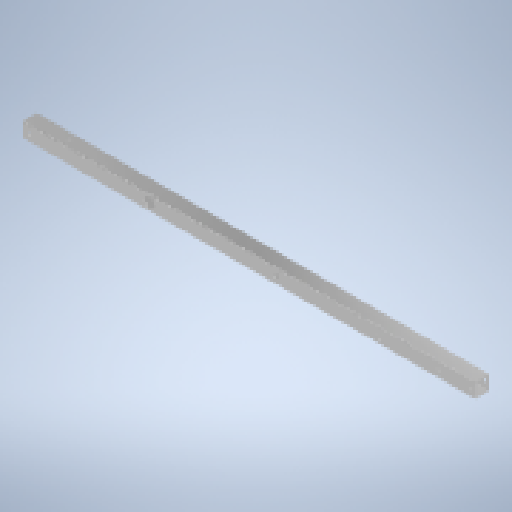
# Autodesk Inventor part: Längs_Traverse_vorne
Saved by Autodesk Inventor 2024.4 (Build 284460000, 460)
## iProperties
Created: 2026-01-10
Part Number: Längs_Traverse_vorne
Material: Aluminium 6061
Description: Längs_Traverse_vorne
Document SubType Name: Modeling
Designer: julia
Mass: 1006.1 g
Surface Area: 3721.63 cm^2
Volume: 372.629 cm^3
Density: 2.7 g/cm^3
Appearance: Aluminium - flach
DocNumber: Längs_Traverse_vorne.ipt
Folder: I60-Konstruktion\I60-Gruppe-7\Gestell\
VDS_Category: Konstruktion
Masse[kg]: 0,377 kg
Autodesk Inventor part; units mm, degrees
ref_plane "YZ Plane" through (0, 0, 0) normal (1, 0, 0) x (0, 1, 0)
ref_plane "XZ Plane" through (0, 0, 0) normal (0, 1, 0) x (-1, 0, 0)
ref_plane "XY Plane" through (0, 0, 0) normal (0, 0, 1) x (1, 0, 0)
sketch "Skizze1" plane through (0, 0, 0) normal (1, 0, 0) x (0, 1, 0)
  line L0 (-19, 20) -> (19, 20)
  line L1 (20, 19) -> (20, -19)
  line L2 (19, -20) -> (-19, -20)
  line L3 (-20, -19) -> (-20, 19)
  line L4 (-20, 20) -> (20, -20) construction
  line L5 (20, 20) -> (-20, -20) construction
  line L6 (-17.5, 18) -> (17.5, 18)
  line L7 (18, 17.5) -> (18, -17.5)
  line L8 (17.5, -18) -> (-17.5, -18)
  line L9 (-18, -17.5) -> (-18, 17.5)
  line L10 (-18, 18) -> (18, -18) construction
  line L11 (18, 18) -> (-18, -18) construction
  arc A0 (20, 19) -> (19, 20) centre (19, 19) ccw
  arc A1 (-19, 20) -> (-20, 19) centre (-19, 19) ccw
  arc A2 (-20, -19) -> (-19, -20) centre (-19, -19) ccw
  arc A3 (19, -20) -> (20, -19) centre (19, -19) ccw
  arc A4 (18, 17.5) -> (17.5, 18) centre (17.5, 17.5) ccw
  arc A5 (-17.5, 18) -> (-18, 17.5) centre (-17.5, 17.5) ccw
  arc A6 (17.5, -18) -> (18, -17.5) centre (17.5, -17.5) ccw
  arc A7 (-18, -17.5) -> (-17.5, -18) centre (-17.5, -17.5) ccw
  point P0 (0, 0)
  dimension "d0" = 40
  dimension "d1" = 40
  dimension "d2" = 36
  dimension "d3" = 36
  dimension "d4" = 1
  dimension "d5" = 0.5
  constraints: 24 end point, 16 point on circle, 16 point on line, 16 tangent, 8 centre point, 5 equal radius, 4 midpoint, 4 parallel, 2 horizontal, 2 perpendicular
  measures "d0" distance of L4.end L5.end
  measures "d1" distance of L5.start L4.end
  measures "d2" distance of L10.end L11.end
  measures "d3" distance of L11.start L10.end
  measures "d4" radius of A0
  measures "d5" radius of A4
extrude "Extrusion1" add sketch "Skizze1" along normal blind 1250
sketch "Skizze2" plane through (0, 20, 19) normal (0, 1, 0) x (1, 0, 0)
  line L0 (0, 19) -> (20, 19)
  line L1 (1250, 38) -> (1250, 0) projected
  line L2 (1250, 19) -> (1150, 19)
  circle A0 centre (1150, 19) radius 5.25
  circle A1 centre (20, 19) radius 5.25
  dimension "d9" = 20
  dimension "d10" = 100
  dimension "d11" = 10.5
  dimension "d12" = 10.5
  constraints: 4 end point, 2 centre point, 2 coincident, 2 horizontal, 1 midpoint
  measures "d9" distance of L0.start L0.end
  measures "d10" distance of L2.start L2.end
  measures "d11" diameter of A0
  measures "d12" diameter of A1
extrude "Extrusion2" cut sketch "Skizze2" against normal blind 1250
sketch "Skizze3" plane through (0, -19, 20) normal (0, 0, 1) x (1, 0, 0)
  line L0 (0, 19) -> (110, 19)
  line L1 (1250, 0) -> (1250, 38) projected
  line L2 (1250, 19) -> (1240, 19)
  circle A0 centre (110, 19) radius 3.2
  dimension "d15" = 110
  dimension "d18" = 6.4
  constraints: 4 end point, 2 horizontal, 1 centre point, 1 coincident, 1 midpoint
  measures "d15" distance of L0.start L0.end
  measures "d18" diameter of A0
extrude "Extrusion3" cut sketch "Skizze3" against normal blind 1250
sketch "Skizze4" plane through (0, -19, 20) normal (0, 0, 1) x (1, 0, 0)
  line L0 (0, 19) -> (110, 19)
  circle A0 centre (110, 19) radius 5.5
  dimension "d21" = 110
  dimension "d22" = 11
  constraints: 2 end point, 1 centre point, 1 coincident, 1 horizontal
  measures "d21" distance of L0.start L0.end
  measures "d22" diameter of A0
extrude "Extrusion4" cut sketch "Skizze4" against normal blind 2
sketch "Skizze6" plane through (0, -20, -19) normal (0, -1, 0) x (1, 0, 0)
  circle A0 centre (1150, 19) radius 5.25 projected
  line L0 (1150, 19) -> (350, 19)
  circle A1 centre (350, 19) radius 14
  point P0 (0, 19)
  dimension "d31" = 800
  dimension "d32" = 28
  constraints: 2 end point, 1 centre point, 1 coincident, 1 horizontal
  measures "d31" distance of L0.start L0.end
  measures "d32" diameter of A1
extrude "Extrusion6" cut sketch "Skizze6" against normal blind 40 contours A1
sketch "Skizze7" plane through (0, 20, 19) normal (0, 1, 0) x (1, 0, 0)
  line L0 (1250, 38) -> (1250, 0) projected
  line L1 (1250, 19) -> (1240, 19)
  circle A0 centre (1240, 19) radius 5.25
  point P0 (0, 19)
  dimension "d35" = 10
  dimension "d36" = 10.5
  constraints: 2 end point, 1 centre point, 1 coincident, 1 horizontal, 1 midpoint
  measures "d35" distance of L1.start L1.end
  measures "d36" diameter of A0
extrude "Extrusion7" cut sketch "Skizze7" against normal through all
sketch "Skizze8" plane through (0, -20, -19) normal (0, -1, 0) x (1, 0, 0)
  line L0 (1250, 1.5) -> (1250, 1) projected
  line L1 (1250, 1) -> (990.0005, 1.5)
  line L2 (0, 1.5) -> (1250, 1.5) projected
  line L3 (990.0005, 1.5) -> (970.0005, 1.5)
  line L4 (0, 0) -> (1250, 0) projected
  line L5 (990.0005, 0) -> (970.0005, 0)
  line L6 (990.0005, 0) -> (990.0005, 20)
  circle A0 centre (990.0005, 20) radius 14
  point P0 (0, 19)
  dimension "d39" = 260
  dimension "d40" = 20
  dimension "d41" = 20
  dimension "d42" = 20
  dimension "d43" = 28
  constraints: 8 end point, 4 point on line, 1 centre point, 1 coincident, 1 perpendicular
  measures "d39" distance of L0.end L1.end
  measures "d40" distance of L1.end L3.end
  measures "d41" distance of L5.start L5.end
  measures "d42" distance of L5.start L6.end
  measures "d43" diameter of A0
extrude "Extrusion8" cut sketch "Skizze8" against normal through all contours A0
sketch "Skizze9" plane through (0, -20, -19) normal (0, -1, 0) x (1, 0, 0)
  line L0 (1250, 1.5) -> (1250, 36.5) projected
  line L1 (1250, 19) -> (700, 19)
  circle A0 centre (700, 19) radius 5.25
  point P0 (0, 19)
  dimension "d46" = 550
  dimension "d47" = 10.5
  constraints: 2 end point, 1 centre point, 1 coincident, 1 horizontal, 1 midpoint
  measures "d46" distance of L1.start L1.end
  measures "d47" diameter of A0
extrude "Extrusion9" cut sketch "Skizze9" against normal through all
